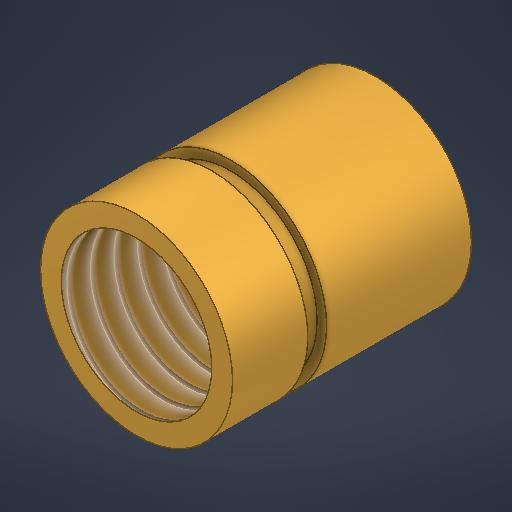
# Autodesk Inventor part: M8-HEATINSERT
Saved by Autodesk Inventor 2025.3 (Build 293356030, 356C)
## iProperties
Created: 2025-10-06
Part Number: M8-HEATINSERT
Material: Generic
Document SubType Name: Modeling
Designer: lstk1ng
Density: 1 g/cm^3
Appearance: Brass - Satin
Author: lstk1ng
Autodesk Inventor part; units mm, degrees
ref_plane "YZ Plane" through (0, 0, 0) normal (1, 0, 0) x (0, 1, 0)
ref_plane "XZ Plane" through (0, 0, 0) normal (0, 1, 0) x (-1, 0, 0)
ref_plane "XY Plane" through (0, 0, 0) normal (0, 0, 1) x (1, 0, 0)
sketch "Sketch1" plane through (0, 0, 0) normal (0, 1, 0) x (-1, 0, 0)
  line L0 (-4, 0) -> (-4, 12.7)
  line L1 (-4, 12.7) -> (-5.1, 12.7)
  line L2 (-4, 0) -> (-5.1, 0)
  line L3 (-5.1, 12.7) -> (-5.1, 8.7)
  line L4 (-5.1, 8.7) -> (-4.6, 8.7)
  line L5 (-4.6, 8.7) -> (-4.6, 7.7)
  line L6 (-4.6, 7.7) -> (-5.1, 7.7)
  line L7 (-5.1, 0) -> (-5.1, 7.7)
  line L8 (-5.1, 8.7) -> (-5.1, 12.7)
  line L9 (0, -2.54) -> (0, 15.24) projected
  point P0 (0, 0)
  dimension "d0" = 5.1
  dimension "d1" = 12.7
  dimension "d2" = 4
  dimension "d3" = 4
  dimension "d4" = 0.5
  dimension "d5" = 1
  constraints: 18 end point, 6 perpendicular, 1 horizontal
  measures "d0" distance of point (0, 0) L2.end
  measures "d1" distance of L2.end L1.end
  measures "d2" distance of point (0, 0) L0.start
  measures "d3" distance of L1.end L3.end
  measures "d4" distance of L3.end L4.end
  measures "d5" distance of L4.end L5.end
revolve "Revolution1" add sketch "Sketch1" angle 360 about axis through (0, 0, -10) along (0, 0, 1)
thread "Thread1" size "M8x1.25" class "6H" standard "ANSI Metric M Profile" length 26.04
body "Solid1"
